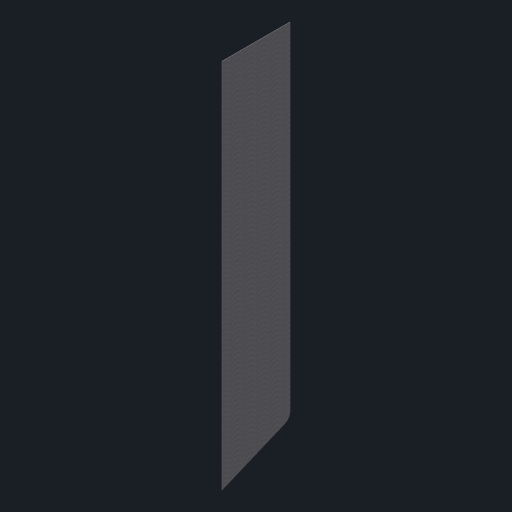
# Autodesk Inventor part: AUX_2._MIRipt
Saved by Autodesk Inventor 2024.3 (Build 283343000, 343)
## iProperties
Created: 2024-07-02
Part Number: AUX_2._MIRipt
Material: Steel, Mild, Welded
Document SubType Name: Modeling
Designer: Niler
Density: 7.85 g/cm^3
Appearance: Weld - Steel Mild
Author: Niler
Autodesk Inventor part; units mm, degrees
ref_plane "YZ Plane" through (0, 0, 0) normal (1, 0, 0) x (0, 1, 0)
ref_plane "XZ Plane" through (0, 0, 0) normal (0, 1, 0) x (-1, 0, 0)
ref_plane "XY Plane" through (0, 0, 0) normal (0, 0, 1) x (1, 0, 0)
sketch "Sketch1" plane through (0, 0, 0) normal (1, 0, 0) x (0, 1, 0)
  line L0 (-512.1922, -107.953) -> (645.1366, -107.953)
  line L1 (645.1366, 125.4929) -> (645.1366, -107.953)
  line L2 (645.1366, 125.4929) -> (-629.4619, 125.4929)
  line L3 (-629.4619, 125.4929) -> (-539.8845, -89.4915)
  arc A0 (-539.8845, -89.4915) -> (-512.1922, -107.953) centre (-512.1922, -77.953) ccw
  point P0 (0, 0)
  constraints: 8 end point, 2 point on circle, 1 centre point
extrude "Extrusion1" add sketch "Sketch1" along normal blind 1.5
body "Solid1"
